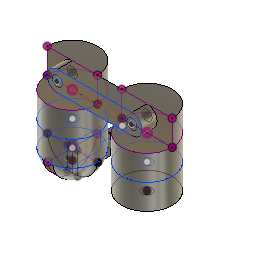
Day17 - Robotic arm part2 (Autodesk Fusion 360 design; units mm, degrees)
Autodesk Fusion 360 part; units mm, degrees
note: some values were not read from the file. Chosen so that the rebuilt part matches the saved one: where a step ends. Set by a fixed rule: which sketch regions a step uses.
sketch "Sketch1" plane through (0, 0, 0) normal (0, 0, 1) x (1, 0, 0) in component "Component"
  circle A0 centre (0, 0) radius 50
  circle A1 centre (0, 0) radius 10
  dimension "d1" = 100
  dimension "d2" = 20
  measures "d1" diameter of A0
  measures "d2" diameter of A1
extrude "Extrude1" add sketch "Sketch1" along normal blind 50 contours A0 | A1 makes body 1 in component "Component"
extrude "Extrude2" add sketch "Sketch1" along normal blind 30 from surface at 50 contours A1 bodies 1 in component "Component"
sketch "Sketch1 (2)" plane through (0, 0, 0) normal (0, 0, 1) x (1, 0, 0) in component "Component'"
  circle A0 centre (-214.7924, -0.6712) radius 50
  circle A1 centre (-214.7924, -0.6712) radius 10
  dimension "d8" = 100
  dimension "d9" = 20
  measures "d8" diameter of A0
  measures "d9" diameter of A1
extrude "Extrude1'" add sketch "Sketch1 (2)" along normal blind 50 separate body makes body 2 in component "Component'"
extrude "Extrude2'" add sketch "Sketch1 (2)" along normal up to surface (20 mm away) from surface at 30 contours A1 bodies 2 in component "Component'"
sketch "Sketch2" plane through (0, 0, 50) normal (0, 0, 1) x (-1, 0, 0) in component "Component'"
  circle A0 centre (214.7924, 0.6712) radius 50
  line L0 (264.7924, 0.6712) -> (164.7924, 0.6712)
extrude "Extrude3" add sketch "Sketch2" along normal blind 50 contours A0 L0 picked at (207.1995, -18.6751) bodies 2 in component "Component'"
sketch "Sketch3" plane through (0, -0.6712, 0) normal (0, -1, 0) x (1, 0, 0) in component "Component'"
  line L0 (-264.7924, 50) -> (-164.7924, 50)
  line L1 (-164.7924, 50) -> (-164.7924, 100)
  line L2 (-164.7924, 100) -> (-264.7924, 100)
  line L3 (-264.7924, 100) -> (-264.7924, 50)
  circle A0 centre (-214.7924, 80) radius 10
  dimension "d17" = 20
  dimension "d18" = 20
  measures "d17" diameter of A0
extrude "Extrude4" add sketch "Sketch3" along normal blind 30 contours A0 bodies 2 in component "Component'"
sketch "Sketch1 (3)" plane through (0, 0, 50) normal (0, 0, 1) x (-1, 0, 0) in component "Component''"
  line L0 (527.8882, 20.1997) -> (379.5594, 20.1997)
  arc A0 (379.5594, 20.1997) -> (379.5594, -19.8003) centre (379.5594, 0.1997) ccw
  line L1 (379.5594, -19.8003) -> (527.8882, -19.8003)
  arc A1 (527.8882, -19.8003) -> (527.8882, 20.1997) centre (527.8882, 0.1997) ccw
  line L2 (527.8882, 0.1997) -> (379.5594, 0.1997) construction
  circle A2 centre (527.8882, 0.1997) radius 10
  circle A3 centre (379.5594, 0.1997) radius 10
  dimension "d21" = 20
  dimension "d23" = 10
  measures "d21" diameter of A2
  measures "d23" distance of A0 A3
extrude "Extrude1''" add sketch "Sketch1 (3)" along normal blind 30 separate body makes body 3 in component "Component''"
sketch "Sketch1 (4)" plane through (0, 0, 0) normal (0, 0, 1) x (1, 0, 0) in component "Component'''"
  circle A0 centre (-221.7811, 2.1941) radius 50
  circle A1 centre (-221.7811, 2.1941) radius 10
  dimension "d8_1" = 100
  dimension "d9_1" = 20
  measures "d8_1" diameter of A0
  measures "d9_1" diameter of A1
extrude "Extrude1'''" add sketch "Sketch1 (4)" along normal blind 50 separate body makes body 4 in component "Component'''"
extrude "Extrude2''" add sketch "Sketch1 (4)" along normal up to surface (20 mm away) from surface at 30 contours A1 bodies 4 in component "Component'''"
sketch "Sketch2 (2)" plane through (0, 0, 50) normal (0, 0, 1) x (-1, 0, 0) in component "Component'''"
  circle A0 centre (221.7811, -2.1941) radius 50
  line L0 (271.7811, -2.1941) -> (171.7811, -2.1941)
extrude "Extrude3'" add sketch "Sketch2 (2)" along normal blind 50 contours A0 L0 picked at (234.7391, -18.4429) bodies 4 in component "Component'''"
sketch "Sketch3 (2)" plane through (0, 2.1941, 0) normal (0, -1, 0) x (1, 0, 0) in component "Component'''"
  line L0 (-271.7811, 50) -> (-171.7811, 50)
  line L1 (-171.7811, 50) -> (-171.7811, 100)
  line L2 (-171.7811, 100) -> (-271.7811, 100)
  line L3 (-271.7811, 100) -> (-271.7811, 50)
  circle A0 centre (-221.7811, 80) radius 10
  dimension "d17_1" = 20
  dimension "d18_1" = 20
  measures "d17_1" diameter of A0
extrude "Extrude4'" add sketch "Sketch3 (2)" along normal blind 30 contours A0 bodies 4 in component "Component'''"
sketch "Sketch1 (5)" plane through (0, 0, 0) normal (0, 0, 1) x (1, 0, 0) in component "Component''''"
  circle A0 centre (282.5375, -0.123) radius 50
  circle A1 centre (282.5375, -0.123) radius 10
  dimension "d86" = 100
  dimension "d87" = 20
  measures "d86" diameter of A0
  measures "d87" diameter of A1
extrude "Extrude1''''" add sketch "Sketch1 (5)" along normal blind 50 separate body contours A0 | A1 makes body 5 in component "Component''''"
extrude "Extrude2'''" add sketch "Sketch1 (5)" along normal blind 30 from surface at 50 contours A1 bodies 5 in component "Component''''"
sketch "Sketch2 (3)" plane through (0, 0, 0) normal (0, 1, 0) x (1, 0, 0) in component "Component''''"
  line L0 (232.5375, 0) -> (332.5375, 0)
  arc A0 (332.5375, 0) -> (232.5375, 0) centre (282.5375, -6.3562) ccw
  line L1 (282.5375, 0) -> (282.5375, 44.0462)
  line L2 (292.5375, 0) -> (292.5375, 44.0462)
  line L3 (272.5375, 0) -> (272.5375, 44.0462)
  dimension "d94" = 10
  dimension "d95" = -10
revolve "Revolve1" add sketch "Sketch2 (3)" angle 360 about axis through (282.5375, 0, 0) along (0, 0, -1) contours L0 A0 L1 L2 | L0 A0 L2 bodies 5 in component "Component''''"
extrude "Extrude3''" cut sketch "Sketch2 (3)" along normal through all and the other way through all contours L0 A0 L1 L3 | L0 A0 L1 L2 bodies 5 in component "Component''''"
ref_plane "WorkPlane1" through (282.5375, 0, -21.5221) normal (-1, 0, 0) x (0, 0, 1) in component "Component''''"
sketch "Sketch3 (3)" plane through (282.5375, 0, -21.5221) normal (-1, 0, 0) x (0, 1, 0) in component "Component''''"
  arc A0 (48.9898, -21.5221) -> (-48.9898, -21.5221) centre (0, -27.8783) ccw
  line L0 (-0.0615, -21.5221) -> (48.9898, -21.5221)
  line L1 (-48.9898, -21.5221) -> (-0.0615, -21.5221)
  circle A1 centre (0, 0) radius 5
  dimension "d97" = 10
  measures "d97" diameter of A1
extrude "Extrude4''" add sketch "Sketch3 (3)" along normal up to far side of body 5 and the other way up to far side of body 5 contours A1 bodies 5 in component "Component''''"
sketch "Sketch1 (6)" plane through (0, 0, 0) normal (0, 0, 1) x (1, 0, 0) in component "Component'''''"
  line L0 (130.9003, 0) -> (130.9003, 65.343)
  line L1 (130.9003, 65.343) -> (170.9003, 65.343)
  line L2 (170.9003, 65.343) -> (170.9003, 0)
  line L3 (130.9003, 0) -> (170.9003, 0)
  circle A0 centre (150.9003, 0) radius 10
  line L4 (150.9003, 0) -> (150.9003, 65.343) construction
  arc A1 (130.9003, 0) -> (170.9003, 0) centre (150.9003, 0) ccw
  line L5 (158.9003, 65.343) -> (142.9003, 65.343)
  line L6 (142.9003, 65.343) -> (142.9003, 98.2557)
  line L7 (142.9003, 98.2557) -> (158.9003, 98.2557)
  line L8 (158.9003, 98.2557) -> (158.9003, 65.343)
  circle A2 centre (150.9003, 109.13) radius 13.5
  circle A3 centre (150.9003, 109.13) radius 10
  dimension "d99" = 20
  dimension "d100" = 40
  dimension "d101" = 16
  dimension "d102" = 27
  dimension "d103" = 20
  measures "d99" diameter of A0
  measures "d102" diameter of A2
  measures "d103" diameter of A3
extrude "Extrude1'''''" add sketch "Sketch1 (6)" along normal blind 20 separate body contours L0 L1 L2 L3 A0 L5 | L3 A0 A1 | L1 L5 L6 L8 A2 | L7 A2 | L7 A2 makes body 6 in component "Component'''''"
component "Component" placed x (1, 0, 0) y (0, 1, 0) z (0, 0, 1) at (0, 0, 0)
component "Component'" placed x (1, 0, 0) y (0, 1, 0) z (0, 0, 1) at (214.7924, 0.6712, 50)
component "Component''" placed x (1, 0, 0) y (0, 0, -1) z (0, 1, 0) at (379.5594, -80, 129.8003)
component "Component'''" placed x (1, 0, 0) y (0, 1, 0) z (0, 0, 1) at (73.4522, -2.1941, 50)
component "Component''''" placed x (1, 0, 0) y (0, 1, 0) z (0, 0, 1) at (-430.8664, 0.123, 0)
component "Component'''''" placed x (0, 0, -1) y (0, 1, 0) z (1, 0, 0) at (-158.3288, 0.123, 129.3782)
